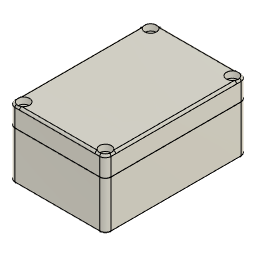
Hộp nhựa 100x68x50mm (Autodesk Fusion 360 design; units mm, degrees)
Autodesk Fusion 360 part; units mm, degrees
sketch "DXF_PCB1_2024-04-22" plane through (0, 0, 0) normal (0, 0, 1) x (1, 0, 0)
  arc A0 (4.4, 24.4) -> (11.4, 24.4) centre (7.9, 24.4) ccw
  arc A1 (11.4, 24.4) -> (4.4, 24.4) centre (7.9, 24.4) ccw
  line L0 (57.4001, 24.4) -> (57.4001, 24.4)
  arc A2 (50.4001, 24.4) -> (57.4001, 24.4) centre (53.9001, 24.4) ccw
  arc A3 (57.4001, 24.4) -> (50.4001, 24.4) centre (53.9001, 24.4) ccw
  arc A4 (11.4, 69.4001) -> (4.4, 69.4001) centre (7.9, 69.4001) ccw
  arc A5 (4.4, 69.4001) -> (11.4, 69.4001) centre (7.9, 69.4001) ccw
  arc A6 (50.4001, 69.4001) -> (57.4001, 69.4001) centre (53.9001, 69.4001) ccw
  arc A7 (57.4001, 69.4001) -> (50.4001, 69.4001) centre (53.9001, 69.4001) ccw
  line L1 (57.4001, 69.4001) -> (57.4001, 69.4001)
  line L2 (34.4001, 6.9) -> (34.4001, 6.9)
  arc A8 (27.4001, 6.9) -> (34.4001, 6.9) centre (30.9001, 6.9) ccw
  arc A9 (34.4001, 6.9) -> (27.4001, 6.9) centre (30.9001, 6.9) ccw
  line L3 (34.4001, 86.9002) -> (34.4001, 86.9002)
  arc A10 (34.4001, 86.9002) -> (27.4001, 86.9002) centre (30.9001, 86.9002) ccw
  arc A11 (27.4001, 86.9002) -> (34.4001, 86.9002) centre (30.9001, 86.9002) ccw
  line L4 (0, 82.9002) -> (0, 10.9)
  arc A12 (10.9, 93.8002) -> (8.9, 91.8002) centre (10.9, 91.8002) ccw
  arc A13 (8.9, 91.8002) -> (2, 84.9002) centre (2, 91.8002) cw
  arc A14 (2, 84.9002) -> (0, 82.9002) centre (2, 82.9002) ccw
  arc A15 (0, 10.9) -> (2, 8.9) centre (2, 10.9) ccw
  arc A16 (2, 8.9) -> (8.9, 2) centre (2, 2) cw
  arc A17 (8.9, 2) -> (10.9, 0) centre (10.9, 2) ccw
  line L5 (10.9, 0) -> (50.9001, 0)
  line L6 (61.8001, 10.9) -> (61.8001, 82.9002)
  arc A18 (50.9001, 0) -> (52.9001, 2) centre (50.9001, 2) ccw
  arc A19 (59.8001, 8.9) -> (61.8001, 10.9) centre (59.8001, 10.9) ccw
  arc A20 (61.8001, 82.9002) -> (59.8001, 84.9002) centre (59.8001, 82.9002) ccw
  arc A21 (52.9001, 2) -> (59.8001, 8.9) centre (59.8001, 2) cw
  arc A22 (52.9001, 91.8002) -> (50.9001, 93.8002) centre (50.9001, 91.8002) ccw
  arc A23 (59.8001, 84.9002) -> (52.9001, 91.8002) centre (59.8001, 91.8002) cw
  line L7 (50.9001, 93.8002) -> (10.9, 93.8002)
  line L8 (0.9001, 96.9) -> (60.9001, 96.9)
  line L9 (64.9001, 92.9) -> (64.9001, 0.9)
  line L10 (60.9001, -3.1) -> (0.9001, -3.1)
  line L11 (-3.0999, 0.9) -> (-3.0999, 92.9)
  circle A24 centre (30.9001, 86.9002) radius 1
  circle A25 centre (7.9, 69.4001) radius 1
  circle A26 centre (53.9001, 69.4001) radius 1
  circle A27 centre (7.9, 24.4) radius 1
  circle A28 centre (30.9001, 6.9) radius 1
  circle A29 centre (53.9001, 24.4) radius 1
  line L12 (-1, 82.9002) -> (-1, 10.9)
  arc A30 (-1, 10.9) -> (2, 7.9) centre (2, 10.9) ccw
  arc A31 (7.9, 2) -> (2, 7.9) centre (2, 2) ccw
  arc A32 (7.9, 2) -> (10.9, -1) centre (10.9, 2) ccw
  line L13 (10.9, -1) -> (50.9001, -1)
  arc A33 (50.9001, -1) -> (53.9001, 2) centre (50.9001, 2) ccw
  arc A34 (59.8001, 7.9) -> (53.9001, 2) centre (59.8001, 2) ccw
  arc A35 (59.8001, 7.9) -> (62.8001, 10.9) centre (59.8001, 10.9) ccw
  line L14 (62.8001, 10.9) -> (62.8001, 82.9002)
  arc A36 (62.8001, 82.9002) -> (59.8001, 85.9002) centre (59.8001, 82.9002) ccw
  arc A37 (53.9001, 91.8002) -> (59.8001, 85.9002) centre (59.8001, 91.8002) ccw
  arc A38 (53.9001, 91.8002) -> (50.9001, 94.8002) centre (50.9001, 91.8002) ccw
  line L15 (50.9001, 94.8002) -> (10.9, 94.8002)
  arc A39 (10.9, 94.8002) -> (7.9, 91.8002) centre (10.9, 91.8002) ccw
  arc A40 (2, 85.9002) -> (7.9, 91.8002) centre (2, 91.8002) ccw
  arc A41 (2, 85.9002) -> (-1, 82.9002) centre (2, 82.9002) ccw
  circle A42 centre (2, 91.8002) radius 2.25
  circle A43 centre (59.8001, 91.8002) radius 2.25
  circle A44 centre (59.8001, 2) radius 2.25
  circle A45 centre (2, 2) radius 2.25
  arc A46 (0.9001, 96.9) -> (-3.0999, 92.9) centre (0.9001, 92.9) ccw
  arc A47 (60.9001, -3.1) -> (64.9001, 0.9) centre (60.9001, 0.9) ccw
  arc A48 (64.9001, 92.9) -> (60.9001, 96.9) centre (60.9001, 92.9) ccw
  arc A49 (-3.0999, 0.9) -> (0.9001, -3.1) centre (0.9001, 0.9) ccw
  circle A50 centre (2, 2) radius 3.4
  circle A51 centre (59.8001, 2) radius 3.4
  circle A52 centre (2, 91.8002) radius 3.4
  circle A53 centre (59.8001, 91.8002) radius 3.4
  circle A54 centre (50.9001, 81.9) radius 2.25
  circle A55 centre (10.9001, 81.9) radius 2.25
  circle A56 centre (50.9001, 11.9) radius 2.25
  circle A57 centre (10.9001, 11.9) radius 2.25
  point P0 (-3.0999, 96.9)
  point P1 (64.9001, 96.9)
  point P2 (-3.0999, -3.1)
  dimension "d1" = 68
  dimension "d2" = 100
  dimension "d5" = 3.1
  dimension "d6" = 3.1
  dimension "d7" = 2
  dimension "d8" = 2
  dimension "d9" = 2
  dimension "d10" = 2
  dimension "d11" = 2
  dimension "d12" = 2
  dimension "d13" = 1
  dimension "d14" = 4.5
  dimension "d15" = 4.5
  dimension "d16" = 4.5
  dimension "d17" = 4.5
  dimension "d18" = 4
  dimension "d27" = 6.8
  dimension "d28" = 6.8
  dimension "d29" = 6.8
  dimension "d30" = 6.8
  dimension "d53" = 4.5
  dimension "d56" = -40
  dimension "d57" = -70
  dimension "d58" = 14
  dimension "d59" = 15
  constraint horizontal L8
  constraint vertical L9
  constraint horizontal L10
  constraint vertical L11
  constraint concentric A10 A24
  constraint concentric A5 A25
  constraint concentric A6 A26
  constraint concentric A0 A27
  constraint concentric A9 A28
  constraint concentric A3 A29
  constraint concentric A13 A42
  constraint concentric A23 A43
  constraint concentric A21 A44
  constraint concentric A16 A45
  constraint coincident P0 L8
  constraint coincident P0 L11
  constraint tangent L8 A46
  constraint tangent L11 A46
  constraint tangent L9 A47
  constraint tangent L10 A47
  constraint equal A46 A47
  constraint coincident P1 L8
  constraint coincident P1 L9
  constraint tangent L8 A48
  constraint tangent L9 A48
  constraint equal A46 A48
  constraint coincident P2 L10
  constraint coincident P2 L11
  constraint tangent L10 A49
  constraint tangent L11 A49
  constraint equal A46 A49
  constraint concentric A16 A50
  constraint concentric A21 A51
  constraint concentric A42 A52
  constraint concentric A23 A53
  measures "d1" distance of P0 P1
  measures "d2" distance of P0 P2
  measures "d5" distance of L5 L10
  measures "d6" distance of L6 L9
  measures "d7" diameter of A24
  measures "d8" diameter of A25
  measures "d9" diameter of A26
  measures "d10" diameter of A27
  measures "d11" diameter of A28
  measures "d12" diameter of A29
  measures "d14" diameter of A42
  measures "d15" diameter of A43
  measures "d16" diameter of A44
  measures "d17" diameter of A45
  measures "d18" radius of A46
  measures "d27" diameter of A50
  measures "d28" diameter of A51
  measures "d29" diameter of A52
  measures "d30" diameter of A53
  measures "d53" diameter of A54
  measures "d58" distance of L9 A54.centre
  measures "d59" distance of L8 A54.centre
extrude "Extrude1" add sketch "DXF_PCB1_2024-04-22" along normal blind 34 contours L8 L9 L10 L11 A46 A47 A48 A49 | A50 | A51 | A52 | A53 makes body 1
extrude "Extrude2" add sketch "DXF_PCB1_2024-04-22" along normal blind 2 separate body contours L4 A12 A13 A14 A15 A16 A17 L5 L6 A18 A19 A20 A21 A22 A23 L7 | A24 | A25 | A26 | A27 | A28 | A29 | A54 | A55 | A56 | A57 makes body 2 at (54.5618, 25.1498, 1.3333) makes body 3 at (24.0886, 40.1936, 0) makes body 4 at (8.8988, 24.3502, 1.3333) makes body 5 at (54.8692, 69.6469, 1.3333) makes body 6 at (31.8691, 87.1469, 1.3333) makes body 7 at (6.9198, 69.5983, 1.3333) makes body 8 at (31.8988, 6.8502, 1.3333)
extrude "Extrude3" add sketch "DXF_PCB1_2024-04-22" along normal blind 35 contours L12 A30 A31 A32 L13 A33 A34 A35 L14 A36 A37 A38 L15 A39 A40 A41 bodies 1 3
extrude "Extrude4" add sketch "DXF_PCB1_2024-04-22" along normal blind 6 contours A0 A1 | A2 A3 | A4 A5 | A6 A7 | A8 A9 | A10 A11 | A54 | A55 | A56 | A57 bodies 1 2 4 5 6 7 8
extrude "Extrude5" cut sketch "DXF_PCB1_2024-04-22" along normal blind 26 contours A50 | A51 | A52 | A53 bodies 1
ref_plane "WorkPlane1" through (30.9001, 46.9, 34.1) normal (0, 0, 1) x (1, 0, 0)
sketch "Sketch2" plane through (0, 0, 34.1) normal (0, 0, 1) x (1, 0, 0)
  arc A0 (53.9001, 91.8002) -> (50.9001, 94.8002) centre (50.9001, 91.8002) ccw construction
  arc A1 (53.9001, 91.8002) -> (59.8001, 85.9002) centre (59.8001, 91.8002) ccw construction
  arc A2 (62.8001, 82.9002) -> (59.8001, 85.9002) centre (59.8001, 82.9002) ccw construction
  line L0 (62.8001, 82.9002) -> (62.8001, 10.9) construction
  arc A3 (59.8001, 7.9) -> (62.8001, 10.9) centre (59.8001, 10.9) ccw construction
  arc A4 (59.8001, 7.9) -> (53.9001, 2) centre (59.8001, 2) ccw construction
  arc A5 (50.9001, -1) -> (53.9001, 2) centre (50.9001, 2) ccw construction
  line L1 (50.9001, -1) -> (10.9, -1) construction
  arc A6 (7.9, 2) -> (10.9, -1) centre (10.9, 2) ccw construction
  arc A7 (7.9, 2) -> (2, 7.9) centre (2, 2) ccw construction
  arc A8 (-1, 10.9) -> (2, 7.9) centre (2, 10.9) ccw construction
  line L2 (-1, 10.9) -> (-1, 82.9002) construction
  arc A9 (2, 85.9002) -> (-1, 82.9002) centre (2, 82.9002) ccw construction
  arc A10 (2, 85.9002) -> (7.9, 91.8002) centre (2, 91.8002) ccw construction
  arc A11 (10.9, 94.8002) -> (7.9, 91.8002) centre (10.9, 91.8002) ccw construction
  line L3 (10.9, 94.8002) -> (50.9001, 94.8002) construction
  circle A12 centre (2, 91.8002) radius 2.25
  circle A13 centre (2, 2) radius 2.25
  circle A14 centre (59.8001, 91.8002) radius 2.25
  circle A15 centre (59.8001, 2) radius 2.25
  arc A16 (0.9001, 96.9) -> (-3.0999, 92.9) centre (0.9001, 92.9) ccw
  line L4 (-3.0999, 92.9) -> (-3.0999, 0.9)
  arc A17 (-3.0999, 0.9) -> (0.9001, -3.1) centre (0.9001, 0.9) ccw
  line L5 (0.9001, -3.1) -> (60.9001, -3.1)
  arc A18 (60.9001, -3.1) -> (64.9001, 0.9) centre (60.9001, 0.9) ccw
  line L6 (64.9001, 0.9) -> (64.9001, 92.9)
  arc A19 (64.9001, 92.9) -> (60.9001, 96.9) centre (60.9001, 92.9) ccw
  line L7 (60.9001, 96.9) -> (0.9001, 96.9)
  arc A20 (59.8001, 10.9) -> (50.9001, 2) centre (59.8001, 2) ccw
  line L8 (59.8001, 82.9002) -> (59.8001, 10.9)
  arc A21 (50.9001, 91.8002) -> (59.8001, 82.9002) centre (59.8001, 91.8002) ccw
  line L9 (10.9, 91.8002) -> (50.9001, 91.8002)
  arc A22 (2, 82.9002) -> (10.9, 91.8002) centre (2, 91.8002) ccw
  line L10 (2, 10.9) -> (2, 82.9002)
  arc A23 (10.9, 2) -> (2, 10.9) centre (2, 2) ccw
  line L11 (50.9001, 2) -> (10.9, 2)
  arc A24 (59.8001, 7.4) -> (63.3001, 10.9) centre (59.8001, 10.9) ccw
  line L12 (63.3001, 82.9002) -> (63.3001, 10.9)
  arc A25 (63.3001, 82.9002) -> (59.8001, 86.4002) centre (59.8001, 82.9002) ccw
  arc A26 (54.4001, 91.8002) -> (59.8001, 86.4002) centre (59.8001, 91.8002) ccw
  arc A27 (54.4001, 91.8002) -> (50.9001, 95.3002) centre (50.9001, 91.8002) ccw
  line L13 (10.9, 95.3002) -> (50.9001, 95.3002)
  arc A28 (10.9, 95.3002) -> (7.4, 91.8002) centre (10.9, 91.8002) ccw
  arc A29 (2, 86.4002) -> (7.4, 91.8002) centre (2, 91.8002) ccw
  arc A30 (2, 86.4002) -> (-1.5, 82.9002) centre (2, 82.9002) ccw
  line L14 (-1.5, 10.9) -> (-1.5, 82.9002)
  arc A31 (-1.5, 10.9) -> (2, 7.4) centre (2, 10.9) ccw
  arc A32 (7.4, 2) -> (2, 7.4) centre (2, 2) ccw
  arc A33 (7.4, 2) -> (10.9, -1.5) centre (10.9, 2) ccw
  line L15 (50.9001, -1.5) -> (10.9, -1.5)
  arc A34 (50.9001, -1.5) -> (54.4001, 2) centre (50.9001, 2) ccw
  arc A35 (59.8001, 7.4) -> (54.4001, 2) centre (59.8001, 2) ccw
  arc A36 (59.8001, 9.9) -> (60.8001, 10.9) centre (59.8001, 10.9) ccw
  line L16 (60.8001, 82.9002) -> (60.8001, 10.9)
  arc A37 (60.8001, 82.9002) -> (59.8001, 83.9002) centre (59.8001, 82.9002) ccw
  arc A38 (51.9001, 91.8002) -> (59.8001, 83.9002) centre (59.8001, 91.8002) ccw
  arc A39 (51.9001, 91.8002) -> (50.9001, 92.8002) centre (50.9001, 91.8002) ccw
  line L17 (10.9, 92.8002) -> (50.9001, 92.8002)
  arc A40 (10.9, 92.8002) -> (9.9, 91.8002) centre (10.9, 91.8002) ccw
  arc A41 (2, 83.9002) -> (9.9, 91.8002) centre (2, 91.8002) ccw
  arc A42 (2, 83.9002) -> (1, 82.9002) centre (2, 82.9002) ccw
  line L18 (1, 10.9) -> (1, 82.9002)
  arc A43 (1, 10.9) -> (2, 9.9) centre (2, 10.9) ccw
  arc A44 (9.9, 2) -> (2, 9.9) centre (2, 2) ccw
  arc A45 (9.9, 2) -> (10.9, 1) centre (10.9, 2) ccw
  line L19 (50.9001, 1) -> (10.9, 1)
  arc A46 (50.9001, 1) -> (51.9001, 2) centre (50.9001, 2) ccw
  arc A47 (59.8001, 9.9) -> (51.9001, 2) centre (59.8001, 2) ccw
  dimension "d34" = 3
  dimension "d35" = -0.5
  dimension "d36" = 2
extrude "Extrude6" add sketch "Sketch2" along normal blind 14 separate body contours A16 L4 A17 L5 A18 L6 A19 L7 | A24 L12 A25 A26 A27 L13 A28 A29 A30 L14 A31 A32 A33 L15 A34 A35 | A36 L16 A37 A38 A39 L17 A40 A41 A42 L18 A43 A44 A45 L19 A46 A47 makes body 9
extrude "Extrude7" cut sketch "Sketch2" along normal blind 3 contours A24 L12 A25 A26 A27 L13 A28 A29 A30 L14 A31 A32 A33 L15 A34 A35 bodies 9
sketch "Sketch3" plane through (0, 0, 48.1) normal (0, 0, 1) x (-1, 0, 0)
  circle A0 centre (-2, -91.8002) radius 2.25
  circle A1 centre (-2, -2) radius 2.25
  circle A2 centre (-59.8001, -91.8002) radius 2.25
  circle A3 centre (-59.8001, -2) radius 2.25
  arc A4 (-59.8001, -10.9) -> (-50.9001, -2) centre (-59.8001, -2) ccw
  line L0 (-50.9001, -2) -> (-10.9, -2)
  arc A5 (-10.9, -2) -> (-2, -10.9) centre (-2, -2) ccw
  line L1 (-2, -10.9) -> (-2, -82.9002)
  arc A6 (-2, -82.9002) -> (-10.9, -91.8002) centre (-2, -91.8002) ccw
  line L2 (-10.9, -91.8002) -> (-50.9001, -91.8002)
  arc A7 (-50.9001, -91.8002) -> (-59.8001, -82.9002) centre (-59.8001, -91.8002) ccw
  line L3 (-59.8001, -82.9002) -> (-59.8001, -10.9)
  line L4 (-60.9001, -96.9) -> (-0.9001, -96.9)
  arc A8 (-0.9001, -96.9) -> (3.0999, -92.9) centre (-0.9001, -92.9) ccw
  line L5 (3.0999, -92.9) -> (3.0999, -0.9)
  arc A9 (3.0999, -0.9) -> (-0.9001, 3.1) centre (-0.9001, -0.9) ccw
  line L6 (-0.9001, 3.1) -> (-60.9001, 3.1)
  arc A10 (-60.9001, 3.1) -> (-64.9001, -0.9) centre (-60.9001, -0.9) ccw
  line L7 (-64.9001, -0.9) -> (-64.9001, -92.9)
  arc A11 (-64.9001, -92.9) -> (-60.9001, -96.9) centre (-60.9001, -92.9) ccw
  circle A12 centre (-59.8001, -2) radius 4.2
  circle A13 centre (-2, -2) radius 4.2
  circle A14 centre (-2, -91.8002) radius 4.2
  circle A15 centre (-59.8001, -91.8002) radius 4.2
  dimension "d41" = 8.4
  dimension "d42" = 8.4
  dimension "d43" = 8.4
  dimension "d44" = 8.4
  constraint concentric A3 A12
  constraint concentric A1 A13
  constraint concentric A0 A14
  constraint concentric A2 A15
  measures "d41" diameter of A12
  measures "d42" diameter of A13
  measures "d43" diameter of A14
  measures "d44" diameter of A15
extrude "Extrude8" add sketch "Sketch3" against normal blind 2 contours A4 L0 A5 L1 A6 L2 A7 L3 bodies 9
extrude "Extrude9" cut sketch "Sketch3" against normal blind 4.5 contours A12 | A13 | A14 | A15 bodies 9
fillet "Fillet1" radius 1.5 8 edges at (64.9001, 46.9, 48.1) (63.7286, 95.7284, 48.1) (30.9001, 96.9, 48.1) (-1.9283, 95.7284, 48.1) (-3.0999, 46.9, 48.1) (-1.9283, -1.9284, 48.1) (30.9001, -3.1, 48.1) (63.7286, -1.9284, 48.1) on bodies 9
fillet "Fillet2" radius 1 8 edges at (63.7286, 95.7284, 0) (64.9001, 46.9, 0) (63.7286, -1.9284, 0) (30.9001, -3.1, 0) (-1.9283, -1.9284, 0) (-3.0999, 46.9, 0) (-1.9283, 95.7284, 0) (30.9001, 96.9, 0) on bodies 1
equation "d58 = ( ( 68 - 40 ) / 2 ) * 1 mm"
equation "d59 = ( ( 100 - 70 ) / 2 ) * 1 mm"
